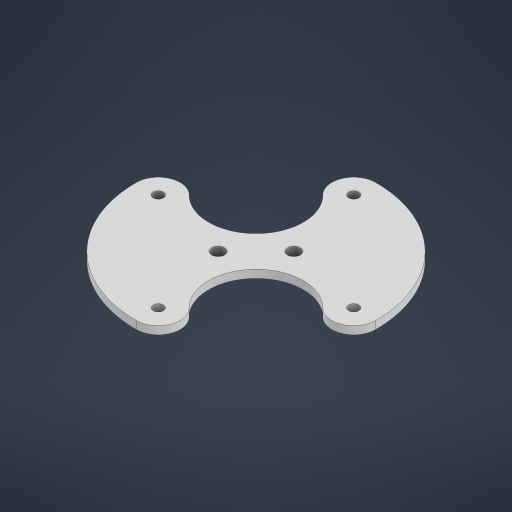
# Autodesk Inventor part: mount-plate
Saved by Autodesk Inventor 2024 (Build 280153000, 153)
## iProperties
Created: 2024-10-06
Part Number: mount-plate
Material: Generic
Document SubType Name: Modeling
Designer: loren
Density: 1 g/cm^3
Appearance: Default
Author: loren
## iProperties of the stored document mount-plate_3DPrint.ipt
Created: 2026-02-06
Part Number: mount-plate_3DPrint
Material: Generic
Document SubType Name: Modeling
Designer: lokies
Density: 1 g/cm^3
Appearance: Default
Author: lokies
Autodesk Inventor part; units mm, degrees
ref_plane "YZ Plane" through (0, 0, 0) normal (1, 0, 0) x (0, 1, 0)
ref_plane "XZ Plane" through (0, 0, 0) normal (0, 1, 0) x (-1, 0, 0)
ref_plane "XY Plane" through (0, 0, 0) normal (0, 0, 1) x (1, 0, 0)
sketch "Sketch2" plane through (0, 0, 0) normal (0, 0, 1) x (1, 0, 0)
  circle A0 centre (6, 6) radius 2
  circle A1 centre (0.0033, 31.0033) radius 1.6
  circle A2 centre (-31.0033, -0.0033) radius 1.6
  line L0 (-31.0033, -0.0033) -> (0.0033, 31.0033) construction
  arc A3 (-26.1066, 4.8934) -> (-4.8934, 26.1066) centre (-15.5, 15.5) ccw
  line L1 (-15.5, 15.5) -> (0, 0) construction
  arc A4 (0.0041, 37.9283) -> (-4.8934, 26.1066) centre (0.0033, 31.0033) ccw
  circle A5 centre (-6, -6) radius 2
  line L2 (6, 6) -> (-6, -6) construction
  arc A6 (26.8194, 26.8194) -> (0.0041, 37.9283) centre (0, 0) ccw
  line L3 (26.8194, 26.8194) -> (7.4142, 7.4142)
  arc A7 (-26.1066, 4.8934) -> (-37.9283, -0.0041) centre (-31.0033, -0.0033) ccw
  arc A8 (-37.9283, -0.0041) -> (-26.8194, -26.8194) centre (0, 0) ccw
  line L4 (-26.8194, -26.8194) -> (-7.4142, -7.4142)
  line L5 (-4.5858, -4.5858) -> (4.5858, 4.5858)
  dimension "d0" = 6
  dimension "d1" = 6
  dimension "d2" = 4
  dimension "d3" = 43.85
  dimension "d4" = 3.2
  dimension "d5" = 30
  dimension "d6" = 15.5
  dimension "d7" = 15.5
  constraints: 14 point on circle, 12 end point, 9 centre point, 5 point on line, 4 coincident, 3 tangent, 2 collinear, 2 equal radius, 2 midpoint, 1 perpendicular
  measures "d0" horizontal distance of L2.start L1.end
  measures "d1" horizontal distance of L2.start L1.end
  measures "d2" diameter of A0
  measures "d3" distance of L0.start L0.end
  measures "d4" diameter of A1
  measures "d5" diameter of A3
  measures "d6" horizontal distance of L1.end L1.start
  measures "d7" horizontal distance of L1.end L1.start
extrude "Extrusion1" add sketch "Sketch2" along normal blind 2.5 contours A0 L5 A5 L4 A8 A7 A3 A4 A6 L3
mirror "Mirror1" about plane through (-4.5858, -4.5858, 0) normal (0.7071, -0.7071, 0)
equation "\"d1\" = d0"
equation "\"d7\" = d6"
body "Solid1"
